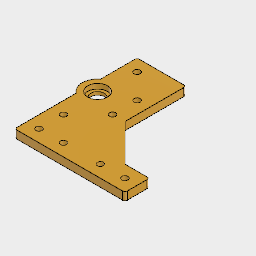
cb_epr (Autodesk Fusion 360 design; units mm, degrees)
Autodesk Fusion 360 part; units mm, degrees
sketch "Sketch1" plane through (0, 0, 0) normal (0, 0, 1) x (1, 0, 0)
  line L0 (39.9557, 100.0182) -> (-0.0443, 100)
  circle A0 centre (9.9956, 10.0044) radius 2.51
  circle A1 centre (29.9956, 10.0044) radius 2.51
  line L1 (39.9589, 50.1826) -> (39.9557, 100.0182)
  line L2 (90, 0.0398) -> (89.9911, 20.0398)
  line L3 (89.9911, 20.0398) -> (70.1185, 20.0382)
  circle A2 centre (79.9956, 10.0354) radius 2.51
  line L4 (-0.031, 70.1204) -> (-0.0443, 100)
  circle A3 centre (29.9576, 50.0136) radius 2.51
  circle A4 centre (9.9602, 30.0045) radius 2.51
  circle A5 centre (9.9602, 90.0045) radius 2.51
  circle A6 centre (7.5583, 60.188) radius 5.5
  circle A7 centre (29.9576, 70.0136) radius 2.51
  line L5 (0, 0) -> (-0.0222, 50.2489)
  line L6 (39.9589, 50.1826) -> (70.1185, 20.0382)
  line L7 (0, 0) -> (90, 0.0398)
  arc A8 (-0.031, 70.1204) -> (-0.0222, 50.2489) centre (7.5583, 60.188) ccw
  circle A9 centre (59.9956, 10.0354) radius 2.51
  dimension "d1" = 100
  dimension "d2" = 90
  dimension "d3" = 5.02
  dimension "d4" = 10
  dimension "d5" = 10
  dimension "d6" = 5.02
  dimension "d7" = 20
  dimension "d8" = 5.02
  dimension "d9" = 5.02
  dimension "d10" = 10
  dimension "d11" = 20
  dimension "d12" = 5.02
  dimension "d13" = 5.02
  dimension "d14" = 5.02
  dimension "d15" = 5.02
  dimension "d16" = 20
  dimension "d18" = 60
  dimension "d19" = 10
  dimension "d20" = 10
  dimension "d21" = 10
  dimension "d22" = 11
  dimension "d23" = 25
  dimension "d24" = 20
  dimension "d33" = 30
  dimension "d35" = 32.4
  dimension "d38" = 40
  dimension "d39" = 10
  dimension "d40" = 30
  constraint coincident L5.start L7.start
  constraint perpendicular L2 L7
  constraint perpendicular L5 L7
  constraint horizontal L5.start L7.start
  constraint concentric A6 A8
  constraint collinear L4 L5
  measures "d1" distance of L5.start
  measures "d2" distance of L5.start
  measures "d3" diameter of A0
  measures "d4" distance of L5.start L7
  measures "d5" distance of L7.start L5
  measures "d6" diameter of A1
  measures "d8" diameter of A2
  measures "d9" diameter of A9
  measures "d10" distance of L2
  measures "d12" diameter of A5
  measures "d13" diameter of A4
  measures "d14" diameter of A3
  measures "d15" diameter of A7
  measures "d19" distance of L7
  measures "d21" distance of L1
  measures "d22" diameter of A6
  measures "d23" diameter of A8
  measures "d33" distance of L5.start L1
  measures "d35" distance of L5.start L1
  measures "d40" distance of L0
extrude "Extrude1" add sketch "Sketch1" along normal blind 6.5
sketch "Sketch4" plane through (0, 0, 6.5) normal (0, 0, 1) x (-1, 0, 0)
  circle A0 centre (-59.9956, -10.0354) radius 2.51
  circle A1 centre (-79.9956, -10.0354) radius 2.51
  circle A2 centre (-29.9956, -10.0044) radius 2.51
  circle A3 centre (-9.9602, -90.0045) radius 2.51
  circle A4 centre (-7.5583, -60.188) radius 5.5
  circle A5 centre (-9.9956, -10.0044) radius 2.51
  circle A6 centre (-29.9576, -70.0136) radius 2.51
  circle A7 centre (-9.9602, -30.0045) radius 2.51
  circle A8 centre (-29.9576, -50.0136) radius 2.51
  line L0 (-39.9589, -50.1826) -> (-39.9557, -100.0182)
  line L1 (-39.9557, -100.0182) -> (0.0443, -100)
  line L2 (0.0443, -100) -> (0.031, -70.1204)
  arc A9 (0.031, -70.1204) -> (0.0222, -50.2489) centre (-7.5583, -60.188) ccw
  line L3 (0.0222, -50.2489) -> (0, 0)
  line L4 (0, 0) -> (-90, -0.0398)
  line L5 (-90, -0.0398) -> (-89.9911, -20.0398)
  line L6 (-89.9911, -20.0398) -> (-70.1185, -20.0382)
  line L7 (-70.1185, -20.0382) -> (-39.9589, -50.1826)
  circle A10 centre (-7.5583, -60.188) radius 8.05
  dimension "d30" = 16.1
  dimension "d37" = 32.4
  constraint concentric A4 A10
  measures "d30" diameter of A10
  measures "d37" distance of L0 L3.end
extrude "Extrude3" cut sketch "Sketch4" against normal blind 4 contours A10
fillet "Fillet1" radius 2 5 edges at (90, 0.0398, 3.25) (89.9911, 20.0398, 3.25) (39.9557, 100.0182, 3.25) (-0.0443, 100, 3.25) (0, 0, 3.25)
